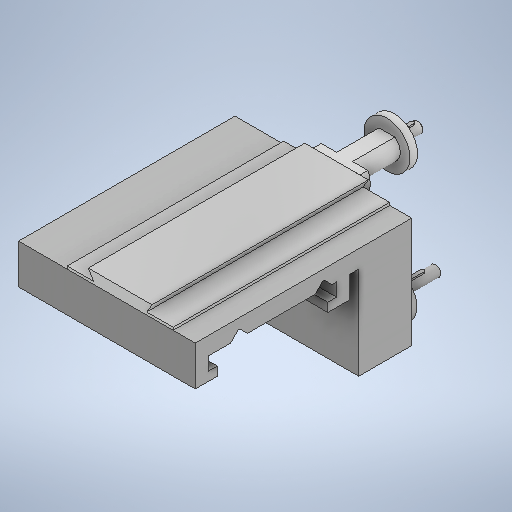
# Autodesk Inventor part: Apron
Saved by Autodesk Inventor 2025 (Build 290162010, 162A)
## iProperties
Created: 2024-08-21
Part Number: Apron
Material: Generic
Document SubType Name: Modeling
Designer: max_d
Density: 1 g/cm^3
Appearance: Default
Author: max_d
Autodesk Inventor part; units mm, degrees
ref_plane "YZ Plane" through (0, 0, 0) normal (1, 0, 0) x (0, 1, 0)
sketch "Sketch1" plane through (0, 0, 0) normal (1, 0, 0) x (0, 1, 0)
  line L0 (0, 0) -> (-105, 0)
  line L1 (-105, 0) -> (-105, -60)
  line L2 (-105, -60) -> (20, -60)
  line L3 (20, -60) -> (20, 185)
  line L4 (20, 185) -> (-15.7857, 185)
  line L5 (0, 145) -> (8.55, 136.45)
  line L6 (8.55, 136.45) -> (8.55, 134.45)
  line L7 (8.55, 134.45) -> (0, 125.9)
  line L8 (0, 125.9) -> (0, 49.35)
  line L9 (0, 49.35) -> (8.55, 40.8)
  line L10 (8.55, 40.8) -> (8.55, 38.8)
  line L11 (8.55, 38.8) -> (0, 30.25)
  line L12 (0, 30.25) -> (0, 25)
  line L13 (0, 25) -> (-15, 25)
  line L14 (-15, 25) -> (-15, 35)
  line L15 (-15, 35) -> (-25, 35)
  line L16 (-25, 35) -> (-25, 10)
  line L17 (-25, 10) -> (0, 10)
  line L18 (0, 10) -> (0, 0)
  line L19 (-25, 160) -> (-25, 185)
  line L20 (-25, 185) -> (-15.7857, 185)
  line L21 (-25, 160) -> (-15, 160)
  line L22 (-15, 160) -> (-15, 170)
  line L23 (-15, 170) -> (0, 170)
  line L24 (0, 170) -> (0, 145)
  line L25 (0, 145) -> (0, 136.45) construction
  line L26 (0, 136.45) -> (8.55, 136.45) construction
  line L27 (0, 125.9) -> (0, 134.45) construction
  line L28 (0, 134.45) -> (8.55, 134.45) construction
  line L29 (0, 49.35) -> (0, 40.8) construction
  line L30 (0, 40.8) -> (8.55, 40.8) construction
  line L31 (0, 30.25) -> (0, 38.8) construction
  line L32 (0, 38.8) -> (8.55, 38.8) construction
  dimension "d0" = 245
  dimension "d1" = 125
  dimension "d2" = 60
  dimension "d3" = 45
  dimension "d4" = 20
  dimension "d5" = 10
  dimension "d6" = 15
  dimension "d7" = 15
  dimension "d8" = 25
  dimension "d9" = 25
  dimension "d10" = 10
  dimension "d11" = 40
  dimension "d14" = 114.75
  dimension "d15" = 2
  dimension "d16" = 8.55
  constraints: 66 end point, 20 perpendicular, 8 point on line, 4 collinear, 3 horizontal, 2 parallel, 1 vertical
  measures "d0" distance of L2.end L3.end
  measures "d1" distance of L1.end L2.end
  measures "d2" distance of L0.end L1.end
  measures "d3" distance between parallel lines of L3 L19
  measures "d4" distance between parallel lines of L3 L8
  measures "d5" distance of L17.end L0.start
  measures "d6" distance between parallel lines of L17 L13
  measures "d7" distance between parallel lines of L4 L23
  measures "d8" distance between parallel lines of L17 L15
  measures "d9" distance of L19.start L19.end
  measures "d10" distance of L19.start L21.end
  measures "d11" distance from line of L4 L5.start
  measures "d14" distance of L11.end L5.start
  measures "d15" distance of L5.end L6.end
  measures "d16" distance between parallel lines of L8 L6
extrude "Extrusion1" add sketch "Sketch1" along normal blind 200
sketch "Sketch2" plane through (0, -105, -60) normal (0, 0, -1) x (-1, 0, 0)
  line L0 (0, 125) -> (-200, 125) projected
  line L1 (-175, 125) -> (-55, 125)
  line L2 (-55, 125) -> (-55, 128)
  line L3 (-55, 128) -> (-175, 128)
  line L4 (-175, 128) -> (-175, 125)
  line L5 (-145, 128) -> (-151, 138)
  line L6 (-151, 138) -> (-79, 138)
  line L7 (-79, 138) -> (-85, 128)
  line L8 (-200, 0) -> (-200, 125) projected
  line L9 (-115, 138) -> (-115, 128) construction
  point P0 (0, 105)
  dimension "d17" = 25
  dimension "d18" = 120
  dimension "d19" = 3
  dimension "d20" = 10
  dimension "d21" = 72
  dimension "d22" = 6
  dimension "d23" = 6
  constraints: 16 end point, 3 point on line, 2 horizontal, 2 midpoint, 2 parallel, 1 perpendicular, 1 vertical
  measures "d17" distance between parallel lines of L8 L4
  measures "d18" distance between parallel lines of L2 L4
  measures "d19" distance of L1.end L2.end
  measures "d20" distance between parallel lines of L6 L3
  measures "d21" distance of L5.end L6.end
  measures "d22" horizontal distance of L6.end L7.end
  measures "d23" horizontal distance of L5.end L5.start
extrude "Extrusion2" add sketch "Sketch2" against normal up to surface (245 mm away) separate body
sketch "Sketch3" plane through (0, -105, -60) normal (0, 0, -1) x (-1, 0, 0)
  line L0 (-150, 85) -> (-80, 85)
  line L1 (-80, 85) -> (-80, 25)
  line L2 (-80, 25) -> (-150, 25)
  line L3 (-150, 25) -> (-150, 85)
  line L4 (-200, 0) -> (-200, 125) projected
  line L5 (0, 0) -> (-200, 0) projected
  point P0 (0, 105)
  dimension "d26" = 70
  dimension "d27" = 60
  dimension "d28" = 50
  dimension "d29" = 25
  constraints: 8 end point, 2 parallel, 1 horizontal, 1 perpendicular
  measures "d26" distance of L0.start L0.end
  measures "d27" distance of L0.end L1.end
  measures "d28" distance between parallel lines of L4 L3
  measures "d29" distance between parallel lines of L5 L2
extrude "Extrusion3" add sketch "Sketch3" along normal blind 35 bodies 1
sketch "Sketch5" plane through (0, -105, -60) normal (0, 0, -1) x (-1, 0, 0)
  circle A0 centre (-115, 126) radius 29
  circle A1 centre (-115, 126) radius 15
  line L0 (-56.8289, 105) -> (-173.1711, 105)
  line L1 (-173.1711, 105) -> (-173.1711, 138)
  line L2 (-173.1711, 138) -> (-56.8289, 138)
  line L3 (-56.8289, 138) -> (-56.8289, 105)
  line L4 (-56.8289, 105) -> (-173.1711, 138) construction
  line L5 (-173.1711, 105) -> (-56.8289, 138) construction
  line L6 (-144.4606, 111) -> (-81.6028, 111) construction
  line L7 (-79, 138) -> (-151, 138) construction
  line L8 (-115, 138) -> (-115, 126) construction
  point P0 (0, 105)
  point P1 (-115, 121.5)
  point P2 (-88.5992, 138)
  point P3 (-106, 138)
  point P4 (-124, 138)
  point P5 (-141.4008, 138)
  point P6 (-135, 105)
  point P7 (-95, 105)
  dimension "d32" = 58
  dimension "d33" = 30
  dimension "d34" = 33
  dimension "d35" = 27
  constraints: 16 end point, 3 midpoint, 2 centre point, 2 horizontal, 2 parallel, 1 coincident, 1 collinear, 1 perpendicular, 1 tangent, 1 vertical, 1 vertical alignment
  measures "d32" diameter of A0
  measures "d33" diameter of A1
  measures "d34" distance of L0.end L1.end
  measures "d35" distance between parallel lines of L2 L6
extrude "Extrusion4" add sketch "Sketch5" along normal blind 9 separate body contours A0 L0 L2 A1
extrude "Extrusion5" add sketch "Sketch5" along normal blind 57 contours A1 L2 picked at (-114.6834, 128.2311) bodies 3
sketch "Sketch6" plane through (0, -105, -117) normal (0, 0, -1) x (-1, 0, 0)
  arc A0 (-124, 138) -> (-106, 138) centre (-115, 126) ccw projected
  circle A1 centre (-115, 126) radius 26
  point P0 (0, 105)
  dimension "d40" = 52
  constraints: 1 centre point, 1 coincident
  measures "d40" diameter of A1
extrude "Extrusion6" add sketch "Sketch6" along normal blind 8.5 bodies 3
sketch "Sketch7" plane through (115, 21, -125.5) normal (0, 0, -1) x (-1, 0, 0)
  circle A0 centre (0, 0) radius 26 projected
  circle A1 centre (0, 0) radius 6
  point P0 (115, -21)
  dimension "d43" = 12
  constraints: 1 centre point, 1 coincident
  measures "d43" diameter of A1
extrude "Extrusion7" add sketch "Sketch7" along normal blind 27 contours A1 bodies 3
sketch "Sketch8" plane through (0, 0, 0) normal (0, 1, 0) x (-1, 0, 0)
  point P0 (0, 0)
ref_plane "Work Plane1" through (115, 27, -125.5) normal (0, 1, 0) x (-1, 0, 0)
sketch "Sketch9" plane through (115, 27, -125.5) normal (0, 1, 0) x (-1, 0, 0)
  line L0 (0, -2) -> (0, -22) construction
  line L1 (-2, -4) -> (-2, -20)
  line L2 (2, -20) -> (2, -4)
  arc A0 (2, -4) -> (-2, -4) centre (0, -4) ccw
  arc A1 (-2, -20) -> (2, -20) centre (0, -20) ccw
  line L3 (-6, -27) -> (6, -27) construction
  line L4 (0, -27) -> (0, -22) construction
  point P0 (115, 125.5)
  point P1 (0, -12)
  point P2 (0, -2)
  dimension "d46" = 4
  dimension "d47" = 20
  dimension "d48" = 5
  constraints: 10 end point, 8 point on circle, 4 tangent, 2 centre point, 2 midpoint, 2 point on line, 2 vertical, 1 parallel
  measures "d46" distance between parallel lines of L2 L1
  measures "d47" distance of L4.end point (0, -2)
  measures "d48" distance of L4.start L4.end
extrude "Extrusion8" add sketch "Sketch9" along normal blind 1.5 and the other way blind 1.25 bodies 3
chamfer "Chamfer1" distance 1 angle 45 1 edges at (121, 21, -152.5)
sketch "Sketch10" plane through (0, -105, -60) normal (0, 0, -1) x (-1, 0, 0)
  circle A0 centre (-175, 35) radius 25
  line L0 (-200, 0) -> (-200, 125) projected
  line L1 (-205.8854, 10) -> (-128.3564, 10) construction
  line L2 (0, 0) -> (-200, 0) construction
  point P0 (0, 105)
  dimension "d56" = 50
  dimension "d57" = 10
  constraints: 2 end point, 2 tangent, 1 centre point, 1 horizontal
  measures "d56" diameter of A0
  measures "d57" distance between parallel lines of L2 L1
extrude "Extrusion9" add sketch "Sketch10" along normal blind 6 bodies 1
sketch "Sketch11" plane through (175, -70, -66) normal (0, 0, -1) x (-1, 0, 0)
  arc A0 (25, 0) -> (-25, 0) centre (0, 0) ccw projected
  circle A1 centre (0, 0) radius 6
  point P0 (175, 70)
  dimension "d60" = 12
  constraints: 1 centre point, 1 coincident
  measures "d60" diameter of A1
extrude "Extrusion10" add sketch "Sketch11" along normal blind 46 bodies 1
ref_plane "Work Plane2" through (175, -64, -66) normal (0, 1, 0) x (-1, 0, 0)
sketch "Sketch12" plane through (175, -64, -66) normal (0, 1, 0) x (-1, 0, 0)
  line L0 (0, -3) -> (0, -33) construction
  line L1 (-2, -5) -> (-2, -31)
  line L2 (2, -31) -> (2, -5)
  arc A0 (2, -5) -> (-2, -5) centre (0, -5) ccw
  arc A1 (-2, -31) -> (2, -31) centre (0, -31) ccw
  line L3 (0, -33) -> (0, -46) construction
  line L4 (-6, -46) -> (6, -46) construction
  point P0 (175, 66)
  point P1 (0, -18)
  point P2 (0, -33)
  point P3 (0, -3)
  dimension "d63" = 4
  dimension "d68" = 30
  dimension "d69" = 13
  constraints: 10 end point, 8 point on circle, 4 tangent, 2 centre point, 2 midpoint, 2 point on line, 2 vertical, 1 parallel
  measures "d63" distance between parallel lines of L1 L2
  measures "d68" distance of point (0, -33) point (0, -3)
  measures "d69" distance of L0.end L3.end
extrude "Extrusion11" add sketch "Sketch12" along normal blind 1.5 and the other way blind 1.5 bodies 1
body "Solid1"
body "Solid2"
body "Solid4"
